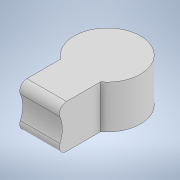
# Autodesk Inventor part: thigh
Saved by Autodesk Inventor 2020.2 (Build 242310000, 310)
## iProperties
Created: 2021-01-29
Part Number: thigh
Material: Generic
Document SubType Name: Modeling
Designer: DELL
Density: 1 g/cm^3
Appearance: Default
Author: DELL
Autodesk Inventor part; units mm, degrees
ref_plane "YZ Plane" through (0, 0, 0) normal (1, 0, 0) x (0, 1, 0)
ref_plane "XZ Plane" through (0, 0, 0) normal (0, 1, 0) x (-1, 0, 0)
ref_plane "UCS1: YZ Plane" through (0, 0, 0) normal (1, 0, 0) x (0, 1, 0)
sketch "Sketch1" plane through (0, 0, 0) normal (1, 0, 0) x (0, 1, 0)
  circle A0 centre (0, 0) radius 30
  line L0 (-30, 0) -> (-30, -130)
  line L1 (-30, -130) -> (30, -130)
  line L2 (30, -130) -> (30, 0)
  circle A1 centre (0, 0) radius 40
  point P0 (30, -26.4575)
  point P1 (-30, -26.4575)
  dimension "d0" = 60
  dimension "d1" = 130
  dimension "d16" = 80
  constraints: 6 end point, 2 centre point, 2 coincident, 2 point on circle, 2 tangent, 2 vertical, 1 perpendicular
  measures "d0" diameter of A0
  measures "d1" distance from line of point (0, 0) L1
  measures "d16" diameter of A1
extrude "Extrusion1" add sketch "Sketch1" along normal mid plane 55 contours L2 L1 L0 A1
sketch "Sketch2" plane through (0, 0, 0) normal (0, 1, 0) x (-1, 0, 0)
  line L0 (27.5, -130) -> (-27.5, -130) projected
  circle A0 centre (0, -130) radius 46
  point P0 (0, 0)
  dimension "d4" = 92
  constraints: 1 centre point, 1 midpoint
  measures "d4" diameter of A0
extrude "Extrusion2" add sketch "Sketch2" along normal mid plane 60
ref_plane "Work Plane1" through (0, 0, -84) normal (0, 0, 1) x (1, 0, 0)
fillet "Fillet1" radius 10 2 edges at (0, 30, -26.4575) (0, -30, -26.4575)
sketch "Sketch3" plane through (0, 0, -84) normal (0, 0, 1) x (1, 0, 0)
  circle A0 centre (0, 0) radius 10
  dimension "d13" = 20
  constraints: 1 centre point, 1 coincident
  measures "d13" diameter of A0
body "Solid1"
